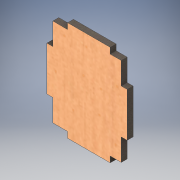
# Autodesk Inventor part: topRL
Saved by Autodesk Inventor 2019 (Build 230136000, 136)
## iProperties
Created: 2020-12-06
Part Number: topRL
Material: Типовые
Document SubType Name: Modeling
Designer: Professional
Density: 1 g/cm^3
Appearance: По умолчанию
Author: Professional
Autodesk Inventor part; units mm, degrees
ref_plane "YZ Plane" through (0, 0, 0) normal (1, 0, 0) x (0, 1, 0)
ref_plane "XZ Plane" through (0, 0, 0) normal (0, 1, 0) x (-1, 0, 0)
ref_plane "XY Plane" through (0, 0, 0) normal (0, 0, 1) x (1, 0, 0)
sketch "Эскиз1" plane through (0, 0, 0) normal (0, 0, 1) x (1, 0, 0)
  line L0 (0, 0) -> (-54.5, 0)
  line L1 (-54.5, 0) -> (-54.5, -15)
  line L2 (-54.5, -15) -> (-50.5, -15)
  line L3 (-50.5, -15) -> (-50.5, -30)
  line L4 (-50.5, -30) -> (-40.5, -30)
  line L5 (-40.5, -30) -> (-40.5, -34)
  line L6 (-40.5, -34) -> (-11.5, -34)
  line L7 (-11.5, -34) -> (-11.5, -30)
  line L8 (-54.5, 0) -> (-54.5, 15)
  line L9 (-54.5, 15) -> (-50.5, 15)
  line L10 (-50.5, 15) -> (-50.5, 30)
  line L11 (-50.5, 30) -> (-40.5, 30)
  line L12 (-40.5, 30) -> (-40.5, 34)
  line L13 (-40.5, 34) -> (-11.5, 34)
  line L14 (-11.5, 34) -> (-11.5, 30)
  line L15 (-11.5, -30) -> (-4, -30)
  line L16 (-4, -30) -> (-4, -15)
  line L17 (-4, -15) -> (0, -15)
  line L18 (0, -15) -> (0, 0)
  line L19 (-11.5, 30) -> (-4, 30)
  line L20 (-4, 30) -> (-4, 15)
  line L21 (-4, 15) -> (0, 15)
  line L22 (0, 15) -> (0, 0)
  dimension "d0" = 29
  dimension "d2" = 10
  dimension "d3" = 30
  dimension "d4" = 15
  dimension "d5" = 4
  dimension "d8" = 11.5
  dimension "d9" = 4
  constraints: 46 end point, 10 symmetric about line, 9 perpendicular, 3 horizontal, 2 equal length, 1 horizontal alignment
  measures "d0" distance of L5.end L6.end
  measures "d2" distance of L3.end L4.end
  measures "d3" diameter of L1.end L0
  measures "d4" distance between parallel lines of L4 L2
  measures "d5" distance of L1.end L2.end
  measures "d8" distance between parallel lines of L7 L18
  measures "d9" distance between parallel lines of L18 L16
extrude "Выдавливание1" add sketch "Эскиз1" along normal blind 4
